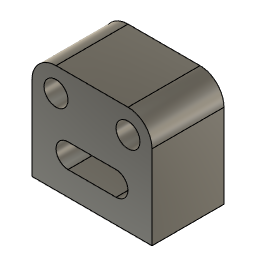
Part 6 (Autodesk Fusion 360 design; units mm, degrees)
Autodesk Fusion 360 part; units mm, degrees
sketch "Sketch5" plane through (0, 0, 0) normal (0, 1, 0) x (1, 0, 0)
  line L0 (50, 30) -> (-50, 30)
  line L1 (-50, 30) -> (-50, -40)
  arc A0 (-50, -40) -> (-30, -60) centre (-30, -40) ccw
  line L2 (-30, -60) -> (30, -60)
  arc A1 (30, -60) -> (50, -40) centre (30, -40) ccw
  line L3 (50, -40) -> (50, 30)
  circle A2 centre (-30, -40) radius 10
  circle A3 centre (30, -40) radius 10
  line L4 (-20, -10) -> (20, -10)
  arc A4 (20, -10) -> (20, 10) centre (20, 0) ccw
  line L5 (20, 10) -> (-20, 10)
  arc A5 (-20, 10) -> (-20, -10) centre (-20, 0) ccw
  line L6 (-30, 0) -> (30, 0) construction
  dimension "d15" = 20
  dimension "d16" = 100
  dimension "d17" = 70
  dimension "d18" = 20
  dimension "d19" = 30
  dimension "d20" = 50
  dimension "d21" = 10
  dimension "d22" = 40
  dimension "d23" = 20
  constraint horizontal L0
  constraint perpendicular L0 L1
  constraint tangent L1 A0
  constraint horizontal L2
  constraint tangent L2 A1
  constraint vertical L3
  constraint tangent A1 L3
  constraint tangent A0 L2
  constraint equal A0 A1
  constraint concentric A0 A2
  constraint concentric A1 A3
  constraint equal A2 A3
  constraint tangent L4 A4
  constraint tangent A4 L5
  constraint parallel L4 L5
  constraint tangent L5 A5
  constraint tangent L4 A5
  constraint midpoint A5 L6.start
  constraint midpoint A4 L6.end
  constraint horizontal L6
  measures "d15" radius of A1
  measures "d16" distance of L0.start L0.end
  measures "d17" distance of L0.start A1.end
  measures "d18" diameter of A2
  measures "d19" distance of origin L0
  measures "d20" distance of origin L1
  measures "d21" radius of A4
  measures "d22" distance of A5.centre A4.centre
  measures "d23" distance of origin A5.centre
extrude "Extrude4" add sketch "Sketch5" along normal blind 60
